Autodesk Fusion 360 part; units mm, degrees
(part 2 of 2)
equation "d125 = ( total_length - ( total_length / 6 ) ) / 2 - wall_distance - material_thickness"
equation "d126 = total_width / 6"
equation "d127 = material_thickness"
equation "d128 = ( total_width - ( total_width / 6 ) ) / 2 - material_thickness - wall_distance"
equation "d130 = total_length / 6"
equation "d132 = total_width / 6"
equation "d133 = material_thickness"
equation "d134 = ( total_width - ( total_width / 6 ) ) / 2 - material_thickness - wall_distance"
equation "d141 = total_width / 6 - 10 mm"
equation "d144 = total_width / 6 - 10 mm"
equation "d145 = -material_thickness"
equation "d150 = bolt_size"
equation "d151 = wall_distance + bolt_size / 2"
equation "d152 = bolt_size"
equation "d153 = wall_distance + bolt_size / 2"
equation "d154 = material_thickness"
equation "d156 = material_thickness"
equation "d158 = bolt_size"
equation "d159 = bolt_size / 2 + wall_distance"
equation "d162 = bolt_size"
equation "d163 = bolt_size / 2"
equation "d164 = material_thickness"
equation "d166 = material_thickness"
equation "d168 = bolt_depth"
equation "d169 = nut_width / 2 - bolt_size / 2"
equation "d170 = nut_thickness"
equation "d171 = nut_width / 2 - bolt_size / 2"
equation "d172 = bolt_size"
equation "d173 = nut_width / 2 - bolt_size / 2"
equation "d174 = nut_thickness"
equation "d175 = nut_width / 2 - bolt_size / 2"
equation "d176 = bolt_depth"
equation "d177 = ( total_width - bolt_size ) / 2"
equation "d179 = bolt_depth / 2"
equation "d180 = bolt_depth"
equation "d181 = nut_width / 2 - bolt_size / 2"
equation "d182 = nut_thickness"
equation "d183 = nut_width / 2 - bolt_size / 2"
equation "d184 = bolt_depth / 2"
equation "d185 = bolt_size"
equation "d186 = bolt_depth / 2"
equation "d187 = nut_width / 2 - bolt_size / 2"
equation "d188 = nut_thickness"
equation "d189 = nut_thickness / 2"
equation "d190 = bolt_depth"
equation "d191 = ( total_width - bolt_size ) / 2"
equation "d192 = pot_holes"
equation "d193 = total_width / 5"
equation "d194 = -material_thickness"
